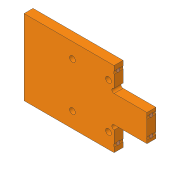
# Autodesk Inventor part: SERVO_MOUNT_TIP
Saved by Autodesk Inventor 2019.4 (Build 234330000, 330)
## iProperties
Created: 2019-11-13
Part Number: SERVO_MOUNT_TIP
Material: 一般
Document SubType Name: Modeling
Designer: y6tada
Density: 1 g/cm^3
Appearance: オレンジ
Mass: 5.91298 g
Surface Area: 39.4688 cm^2
Volume: 5.91298 cm^3
Author: y6tada
Autodesk Inventor part; units mm, degrees
ref_plane "YZ Plane" through (0, 0, 0) normal (1, 0, 0) x (0, 1, 0)
ref_plane "XZ Plane" through (0, 0, 0) normal (0, 1, 0) x (-1, 0, 0)
ref_plane "XY Plane" through (0, 0, 0) normal (0, 0, 1) x (1, 0, 0)
sketch "スケッチ1" plane through (0, 0, 0) normal (0, 0, 1) x (1, 0, 0)
  line L0 (14, 10) -> (30, 10) construction
  line L1 (30, 10) -> (30, -10) construction
  line L2 (30, -10) -> (14, -10) construction
  line L3 (14, -10) -> (14, 10) construction
  line L4 (0, 0) -> (42.5052, 0) construction
  line L5 (-7.5, 16.75) -> (32.5, 16.75)
  line L6 (47.1, 6) -> (47.1, 4.6)
  line L7 (32.5, -16.75) -> (-7.5, -16.75)
  line L8 (32.5, 16.75) -> (32.5, 14.6)
  line L9 (32.5, 8) -> (32.5, 6) construction
  line L10 (32.5, 6) -> (47.1, 6)
  arc A0 (32.5, 8) -> (32.5, 6) centre (32.5, 7) ccw
  line L11 (32.5, -16.75) -> (32.5, -14.6)
  line L12 (32.5, -6) -> (47.1, -6)
  arc A1 (32.5, -6) -> (32.5, -8) centre (32.5, -7) ccw
  line L13 (32.5, 6) -> (32.5, -6) construction
  line L14 (32.5, -8) -> (32.5, -6) construction
  arc A2 (47.1, 4.6) -> (47.1, 3.4) centre (47.9, 4) ccw
  arc A3 (47.1, -3.4) -> (47.1, -4.6) centre (47.9, -4) ccw
  line L15 (47.1, 4.6) -> (47.1, 3.4) construction
  line L16 (47.1, 3.4) -> (47.1, -3.4)
  line L17 (47.1, -3.4) -> (47.1, -4.6) construction
  line L18 (47.1, -4.6) -> (47.1, -6)
  arc A4 (32.5, 14.6) -> (32.5, 13.4) centre (33.3, 14) ccw
  line L19 (32.5, 13.4) -> (32.5, 8)
  line L20 (32.5, 14.6) -> (32.5, 13.4) construction
  line L21 (33.7, 6) -> (33.7, -6) construction
  arc A5 (32.5, -13.4) -> (32.5, -14.6) centre (33.3, -14) ccw
  line L22 (32.5, -13.4) -> (32.5, -8)
  line L23 (32.5, -14.6) -> (32.5, -13.4) construction
  line L24 (-7.5, 16.75) -> (-7.5, -16.75)
  line L25 (35.7, 6) -> (35.7, -6) construction
  dimension "d0" = 20
  dimension "d1" = 16
  dimension "d3" = 1
  dimension "d4" = 12
  dimension "d5" = 2.5
  dimension "d7" = 1
  dimension "d8" = 0.8
  dimension "d9" = 8
  dimension "d10" = 0.8
  dimension "d11" = 28
  dimension "d12" = 33.5
  dimension "d29" = 1.2
  dimension "d32" = 40
  dimension "d34" = 32.5
  dimension "d36" = 2
  dimension "d37" = 11.4
  constraints: 52 end point, 14 perpendicular, 12 point on circle, 11 symmetric about line, 6 centre point, 5 parallel, 4 coincident, 3 horizontal, 3 point on line, 2 vertical, 1 collinear, 1 equal radius, 1 tangent, 5 other
  measures "d0" distance of L0.end L1.end
  measures "d1" distance of L0.start L0.end
  measures "d3" radius of A0
  measures "d4" diameter of L10 L4
  measures "d5" distance between parallel lines of L8 L1
  measures "d7" radius of A2
  measures "d8" distance from line of L6 A2.centre
  measures "d9" diameter of A2.centre L4
  measures "d10" distance from line of L8 A4.centre
  measures "d11" diameter of A4.centre L4
  measures "d12" distance between parallel lines of L7 L5
  measures "d29" distance between parallel lines of L13 L21
  measures "d32" distance between parallel lines of L19 L24
  measures "d34" distance from line of L4.start L19
  measures "d36" distance between parallel lines of L21 L25
  measures "d37" distance between parallel lines of L16 L25
extrude "押し出し1" add sketch "スケッチ1" along normal blind 4
hole "穴1" at (14, 10, 0) at (30, 10, 0) at (30, -10, 0) at (14, -10, 0) direction (0, 0, 1) diameter 2.6 end through all clearance for "Countersunk Raised Head Screw ISO 2010/7047" size "M2.5" standard "ISO"
sketch "スケッチ2" plane through (32.5, 8, 0) normal (1, 0, 0) x (0, 0, -1)
  line L0 (0, 6.6) -> (-4, 6.6) construction
  line L1 (0, 5.4) -> (-4, 5.4) construction
  line L2 (-4, 6.6) -> (0, 5.4) construction
  line L3 (0, -21.4) -> (-4, -21.4) construction
  line L4 (0, -22.6) -> (-4, -22.6) construction
  line L5 (-4, -21.4) -> (0, -22.6) construction
  point P0 (0, -8)
  point P1 (-2, 6)
  point P2 (-2, -22)
  constraints: 4 end point, 2 midpoint
hole "穴2" at (32.5, 14, 2) at (32.5, -14, 2) direction (-1, 0, 0) diameter 1.567 depth 6 tip angle 118 thread size "M2x0.4" class "6H" standard "ISO Metric profile"
sketch "スケッチ3" plane through (47.1, -3.4, 0) normal (1, 0, 0) x (0, 0, -1)
  line L0 (0, -1.2) -> (-4, -1.2) construction
  line L1 (0, 0) -> (-4, 0) construction
  line L2 (0, -1.2) -> (-4, 0) construction
  line L3 (0, 6.8) -> (-4, 6.8) construction
  line L4 (0, 8) -> (-4, 8) construction
  line L5 (0, 6.8) -> (-4, 8) construction
  point P0 (0, 3.4)
  point P1 (-2, -0.6)
  point P2 (-2, 7.4)
  constraints: 4 end point, 2 midpoint
hole "穴3" at (47.1, -4, 2) at (47.1, 4, 2) direction (-1, 0, 0) diameter 1.567 depth 6.3 tip angle 118 thread size "M2x0.4" class "6H" standard "ISO Metric profile"
